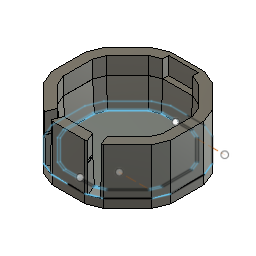
Lens Cap (Autodesk Fusion 360 design; units mm, degrees)
Autodesk Fusion 360 part; units mm, degrees
note: some values were not read from the file. Chosen so that the rebuilt part matches the saved one: which face or edge a step refers to; which pieces of a blend or face edit are solid.
sketch "Sketch1" plane through (0, 0, 0) normal (0, 1, 0) x (1, 0, 0)
  line L0 (0, 16.5) -> (5, 16.5)
  line L1 (0, -16.5) -> (4.9, -16.5)
  line L2 (16.5, 4.9) -> (16.5, -5)
  line L3 (8.1673, 15.1673) -> (15.2383, 8.0962)
  line L4 (8.1673, 15.1673) -> (18.1673, 15.1673) construction
  line L5 (15.1673, -8.1673) -> (8.0962, -15.2383)
  line L6 (15.1673, -8.1673) -> (5.1673, -8.1673) construction
  line L7 (16.5, -5) -> (15.1673, -8.1673)
  line L8 (8.0962, -15.2383) -> (4.9, -16.5)
  line L9 (16.5, 4.9) -> (15.2383, 8.0962)
  line L10 (8.1673, 15.1673) -> (5, 16.5)
  line L11 (0, 16.5) -> (-5, 16.5)
  line L12 (-8.1673, 15.1673) -> (-5, 16.5)
  line L13 (-8.1673, 15.1673) -> (-15.2383, 8.0962)
  line L14 (-16.5, 4.9) -> (-15.2383, 8.0962)
  line L15 (-16.5, 4.9) -> (-16.5, -5)
  line L16 (-16.5, -5) -> (-15.1673, -8.1673)
  line L17 (-15.1673, -8.1673) -> (-8.0962, -15.2383)
  line L18 (-8.0962, -15.2383) -> (-4.9, -16.5)
  line L19 (0, -16.5) -> (-4.9, -16.5)
  line L20 (10.3374, -18.654) -> (5.6609, -20.5)
  line L21 (0, -20.5) -> (5.6609, -20.5)
  line L22 (0, -20.5) -> (-5.6609, -20.5)
  line L23 (-10.3374, -18.654) -> (-5.6609, -20.5)
  line L24 (-18.5501, -10.4413) -> (-10.3374, -18.654)
  line L25 (-20.5, -5.8073) -> (-18.5501, -10.4413)
  line L26 (-20.5, 5.6609) -> (-20.5, -5.8073)
  line L27 (-20.5, 5.6609) -> (-18.654, 10.3374)
  line L28 (-10.4413, 18.5501) -> (-18.654, 10.3374)
  line L29 (-10.4413, 18.5501) -> (-5.8073, 20.5)
  line L30 (0, 20.5) -> (-5.8073, 20.5)
  line L31 (0, 20.5) -> (5.8073, 20.5)
  line L32 (10.4413, 18.5501) -> (5.8073, 20.5)
  line L33 (10.4413, 18.5501) -> (18.654, 10.3374)
  line L34 (20.5, 5.6609) -> (18.654, 10.3374)
  line L35 (20.5, 5.6609) -> (20.5, -5.8073)
  line L36 (20.5, -5.8073) -> (18.5501, -10.4413)
  line L37 (18.5501, -10.4413) -> (10.3374, -18.654)
  line L38 (0, -17.15) -> (5.0236, -17.15)
  line L39 (8.4604, -15.7934) -> (5.0236, -17.15)
  line L40 (15.717, -8.5368) -> (8.4604, -15.7934)
  line L41 (17.15, -5.1312) -> (15.717, -8.5368)
  line L42 (17.15, 5.0236) -> (17.15, -5.1312)
  line L43 (17.15, 5.0236) -> (15.7934, 8.4604)
  line L44 (8.5368, 15.717) -> (15.7934, 8.4604)
  line L45 (8.5368, 15.717) -> (5.1312, 17.15)
  line L46 (0, 17.15) -> (5.1312, 17.15)
  line L47 (0, 17.15) -> (-5.1312, 17.15)
  line L48 (-8.5368, 15.717) -> (-5.1312, 17.15)
  line L49 (-8.5368, 15.717) -> (-15.7934, 8.4604)
  line L50 (-17.15, 5.0236) -> (-15.7934, 8.4604)
  line L51 (-17.15, 5.0236) -> (-17.15, -5.1312)
  line L52 (-17.15, -5.1312) -> (-15.717, -8.5368)
  line L53 (-15.717, -8.5368) -> (-8.4604, -15.7934)
  line L54 (-8.4604, -15.7934) -> (-5.0236, -17.15)
  line L55 (0, -17.15) -> (-5.0236, -17.15)
  dimension "d1" = 16.5
  dimension "d2" = 16.5
  dimension "d4" = 16.5
  dimension "d5" = 10
  dimension "d6" = 45
  dimension "d7" = 16.5
  dimension "d8" = 45
  dimension "d9" = 10
  dimension "d10" = 16.5
  dimension "d11" = 4
  dimension "d45" = 0.65
  constraint horizontal L0
  constraint horizontal L1
  constraint vertical L2
  constraint horizontal L4
  constraint horizontal L6
  constraint equal L7 L8
  constraint equal L9 L10
  measures "d1" distance of origin L0
  measures "d2" distance of origin L1
  measures "d4" distance of origin L2
  measures "d5" distance of L3.start L3.end
  measures "d6" angle of L3 L4
  measures "d7" distance of origin L3
  measures "d8" angle of L5 L6
  measures "d9" distance of L5.start L5.end
  measures "d10" distance of origin L5
extrude "Extrude13" add sketch "Sketch1" against normal blind 3 contours L0 L1 L2 L3 L5 L7 L8 L9 L10 L11 L12 L13 L14 L15 L16 L17 L18 L19 | L20 L21 L22 L23 L24 L25 L26 L27 L28 L29 L30 L31 L32 L33 L34 L35 L36 L37 | L38 L39 L40 L41 L42 L43 L44 L45 L46 L47 L48 L49 L50 L51 L52 L53 L54 L55
extrude "Extrude14" add sketch "Sketch1" along normal blind 16 contours L20 L21 L22 L23 L24 L25 L26 L27 L28 L29 L30 L31 L32 L33 L34 L35 L36 L37
extrude "Extrude15" add sketch "Sketch1" along normal blind 10 contours L38 L39 L40 L41 L42 L43 L44 L45 L46 L47 L48 L49 L50 L51 L52 L53 L54 L55
draft "Draft2" angle 4 neutral plane through (0, 0, 0) pull (0, 1, 0) 16 faces at (10.5243, 3.3333, -12.8102) (16.0794, 3.3333, -5.9654) (16.5, 3.3333, -1.6) (16.0558, 3.3333, 6.0558) (7.1115, 3.3333, -15.6115) (1.6667, 3.3333, -16.5) (-7.1115, 3.3333, -15.6115) (-10.5243, 3.3333, -12.8102) (-16.0794, 3.3333, -5.9654) (-16.5, 3.3333, -1.6) (-16.0558, 3.3333, 6.0558) (-12.8102, 3.3333, 10.5243) (-7.0308, 3.3333, 15.6589) (-1.6333, 3.3333, 16.5) (7.0308, 3.3333, 15.6589) (12.8102, 3.3333, 10.5243)
extrude "Extrude16" cut 1 faces at (-1.7104, 12, -17.15) along direction (0, 0, -1) blind 2
extrude "Extrude17" add 1 faces at (-1.6745, 12, 17.15) along direction (0, 0, -1) blind 1
chamfer "Chamfer6" distance 1 angle 45 4 edges at (0, 16, 16.15) (5.0236, 13, 16.15) (0, 10, 16.15) (-5.0236, 13, 16.15)
extrude "Extrude18" cut 1 faces at (7.3148, 12, 16.2456) along direction (0.367166, 0, 0.930155) blind 4
extrude "Extrude19" cut 1 faces at (7.2055, 6.6667, 16.0911) along direction (0.366272, -0.069756, 0.92789) blind 4
extrude "Extrude20" cut 1 faces at (-7.2057, 6.6667, 16.091) along direction (-0.366272, -0.069756, 0.92789) blind 7
extrude "Extrude21" cut 1 faces at (-7.3148, 12, 16.2456) along direction (-0.367166, 0, 0.930155) blind 5
extrude "Extrude22" cut 1 faces at (-6.9952, 10, 18.7904) along direction (0, -1, 0) blind 1
extrude "Extrude23" cut 1 faces at (8.1408, 10, 18.3382) along direction (0, -1, 0) blind 1
equation "d1 = ( 33 / 2 ) * 1 mm"
equation "d2 = ( 33 / 2 ) * 1 mm"
equation "d8 = 90 deg - 45 deg"
